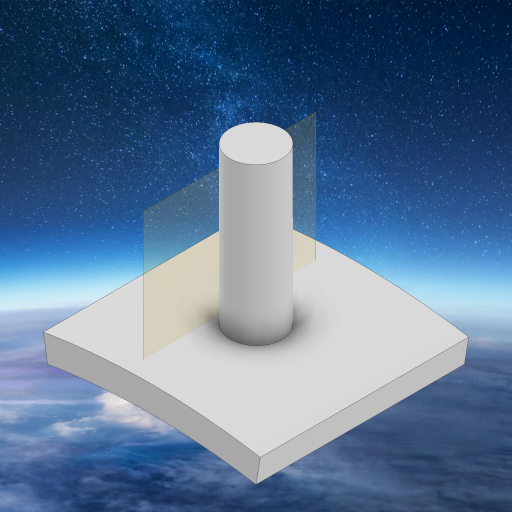
# Autodesk Inventor part: shiftt_fixed_plate2
Saved by Autodesk Inventor 2023 (Build 270158000, 158)
## iProperties
Created: 2023-10-24
Part Number: shiftt_fixed_plate2
Material: 一般
Document SubType Name: Modeling
Designer: 310611102
Density: 1 g/cm^3
Appearance: 預設
Author: 310611102
Autodesk Inventor part; units mm, degrees
ref_plane "XY Plane" through (0, 0, 0) normal (0, 0, 1) x (1, 0, 0)
sketch "Sketch1" plane through (0, 0, 0) normal (0, 0, 1) x (1, 0, 0)
  arc A0 (20.8333, 123.2517) -> (-20.8333, 123.2517) centre (0, 0) ccw
  arc A1 (20, 118.3216) -> (-20, 118.3216) centre (0, 0) ccw
  line L0 (0, 0) -> (0, 143.8844) construction
  line L1 (-20, 118.3216) -> (-20.8333, 123.2517)
  line L2 (20, 118.3216) -> (20.8333, 123.2517)
  dimension "d0" = 250
  dimension "d1" = 5
  dimension "d2" = 40
  constraints: 6 end point, 4 point on circle, 2 centre point, 2 symmetric about line, 1 coincident, 1 line through centre, 1 vertical
  measures "d0" diameter of A0
  measures "d1" radial gap between concentric circles of A0 A1
  measures "d2" distance of L2.start L1.start
extrude "Extrusion1" add sketch "Sketch1" along normal mid plane 40
ref_plane "Work Plane1" through (0, 120, 0) normal (0, 1, 0) x (-1, 0, 0)
sketch "Sketch2" plane through (0, 120, 0) normal (0, 1, 0) x (-1, 0, 0)
  circle A0 centre (0, 0) radius 5
  point P0 (0, 0)
  dimension "d5" = 10
  constraints: 1 centre point, 1 coincident
  measures "d5" diameter of A0
extrude "Extrusion2" add sketch "Sketch2" along normal blind 35
ref_plane "Work Plane2" through (-5, 120, 0) normal (1, 0, 0) x (0, 1, 0)
sketch "Sketch3" plane through (-5, 120, 0) normal (1, 0, 0) x (0, 1, 0)
  circle A0 centre (30, 0) radius 1.8
  line L0 (35, -5) -> (35, 5) projected
  line L1 (-151, 0) -> (66, 0) projected
  point P0 (-120, 0)
  dimension "d8" = 3.6
  dimension "d9" = 5
  constraints: 1 centre point, 1 point on line
  measures "d8" diameter of A0
  measures "d9" distance from line of L0 A0.centre
extrude "Extrusion3" cut sketch "Sketch3" along normal blind 5
chamfer "Chamfer1" distance 0.5 angle 45 2 edges at (-4.6648, 149.9993, -1.8) (-4.6648, 150.0007, 1.8)
body "Solid1"
